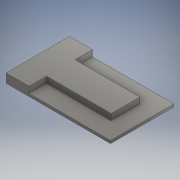
# Autodesk Inventor part: Base
Saved by Autodesk Inventor 2018 (Build 220112000, 112)
## iProperties
Created: 2020-09-24
Part Number: Base
Material: Stainless Steel
Document SubType Name: Modeling
Designer: supervisor
Density: 8 g/cm^3
Appearance: Semi-Polished
Author: supervisor
Autodesk Inventor part; units mm, degrees
ref_plane "YZ Plane" through (0, 0, 0) normal (1, 0, 0) x (0, 1, 0)
ref_plane "XZ Plane" through (0, 0, 0) normal (0, 1, 0) x (-1, 0, 0)
ref_plane "XY Plane" through (0, 0, 0) normal (0, 0, 1) x (1, 0, 0)
sketch "Sketch1" plane through (0, 0, 0) normal (0, 0, 1) x (1, 0, 0)
  line L0 (0, 0) -> (150, 0)
  line L1 (150, 0) -> (150, 91)
  line L2 (150, 91) -> (0, 91)
  line L3 (0, 91) -> (0, 0)
  dimension "d0" = 150
  dimension "d1" = 91
  constraints: 8 end point, 2 parallel, 1 horizontal, 1 perpendicular
  measures "d0" distance of L1.end L2.end
  measures "d1" distance of L2.end L0.start
extrude "Extrusion1" add sketch "Sketch1" along normal blind 13
sketch "Sketch2" plane through (0, 0, 13) normal (0, 0, 1) x (1, 0, 0)
  line L0 (150, 0) -> (150, 91) projected
  line L1 (150, 91) -> (33, 91)
  line L2 (33, 91) -> (33, 66)
  line L3 (33, 66) -> (150, 66)
  line L4 (150, 66) -> (150, 91)
  line L5 (0, 0) -> (150, 0) projected
  line L6 (150, 0) -> (33, 0)
  line L7 (33, 0) -> (33, 25)
  line L8 (33, 25) -> (150, 25)
  line L9 (150, 25) -> (150, 0)
  dimension "d4" = 25
  dimension "d5" = 25
  dimension "d6" = 117
  dimension "d7" = 117
  constraints: 16 end point, 4 parallel, 2 horizontal, 2 perpendicular
  measures "d4" distance of L6.end L7.end
  measures "d5" distance of L1.end L2.end
  measures "d6" distance between parallel lines of L2 L0
  measures "d7" distance of L7.end L8.end
extrude "Extrusion2" cut sketch "Sketch2" against normal blind 9
sketch "Sketch3" plane through (0, 0, 0) normal (0, 0, -1) x (-1, 0, 0)
  line L0 (-150, 66) -> (-33, 66) projected
  line L1 (-33, 25) -> (-150, 25) projected
  line L2 (-33, 66) -> (-33, 91) projected
  line L3 (0, 91) -> (0, 0) projected
  line L4 (-150, 91) -> (0, 91) projected
  line L5 (0, 0) -> (-150, 0) projected
  line L6 (-33, 0) -> (-33, 25) projected
  line L7 (-124, 63) -> (-5, 63)
  line L8 (-5, 63) -> (-5, 28)
  line L9 (-5, 28) -> (-124, 28)
  line L10 (-124, 28) -> (-124, 63)
  line L11 (-150, 0) -> (-150, 91) projected
  dimension "d10" = 3
  dimension "d11" = 3
  dimension "d12" = 5
  dimension "d16" = 26
  constraints: 8 end point, 2 parallel, 1 horizontal, 1 perpendicular
  measures "d10" distance between parallel lines of L7 L0
  measures "d11" distance between parallel lines of L1 L9
  measures "d12" distance between parallel lines of L8 L3
  measures "d16" distance between parallel lines of L11 L10
extrude "Extrusion3" cut sketch "Sketch3" against normal blind 10 contours L7 L8 L9 L10
sketch "Sketch4" plane through (0, 0, 13) normal (0, 0, 1) x (1, 0, 0)
  line L0 (150, 66) -> (126, 66)
  line L1 (126, 66) -> (126, 25)
  line L2 (126, 25) -> (150, 25)
  line L3 (150, 25) -> (150, 66)
  line L4 (33, 25) -> (150, 25) projected
  line L5 (150, 66) -> (33, 66) projected
  line L6 (150, 25) -> (150, 66) projected
  point P0 (0, 0)
  dimension "d17" = 24
  constraints: 8 end point, 3 collinear, 2 parallel, 1 horizontal, 1 perpendicular
  measures "d17" distance between parallel lines of L1 L3
extrude "Extrusion4" cut sketch "Sketch4" against normal blind 9
equation "\"d11\" = d10"
body "Solid1"
